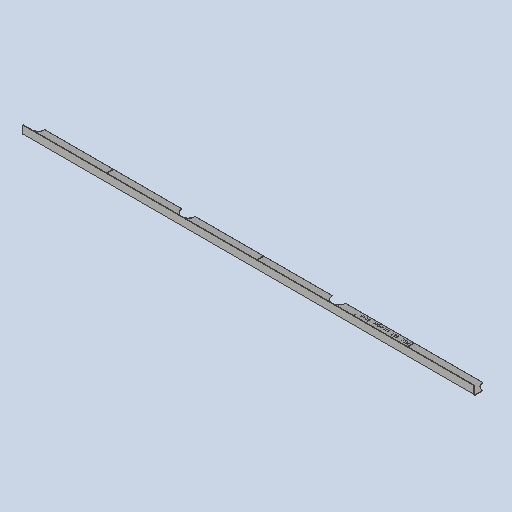
# Autodesk Inventor part: MSC 061 stringer back ^
Saved by Autodesk Inventor 2024.2 (Build 282272000, 272)
## iProperties
Created: 2024-04-28
Part Number: MSC 061 stringer back ^
Material: Stainless Steel
Document SubType Name: Sheet Metal
Designer: pokla
Density: 8 g/cm^3
Sheet Metal Rule: AISI304 2mm Die16
Appearance: Default
Flat Pattern Width: 150 cm
Flat Pattern Length: 7.7967 cm
Flat Pattern Area: 1169.51 cm^2
Sheet Metal Width: 1500,000 mm
Sheet Metal Length: 77,967 mm
Sheet Metal Area: 116950,534 mm^2
Stock Number: МОО 061 стрингер спина ^
Author: admin
Autodesk Inventor part; units mm, degrees
ref_plane "YZ Plane" through (0, 0, 0) normal (1, 0, 0) x (0, 1, 0)
ref_plane "XZ Plane" through (0, 0, 0) normal (0, 1, 0) x (-1, 0, 0)
ref_plane "XY Plane" through (0, 0, 0) normal (0, 0, 1) x (1, 0, 0)
sketch "Sketch1" plane through (0, 0, 0) normal (0, 0, 1) x (1, 0, 0)
  line L0 (-750, 51.765) -> (750, 51.765)
  line L1 (750, 51.765) -> (750, 0)
  line L2 (750, 0) -> (-750, 0)
  line L3 (-750, 0) -> (-750, 51.765)
  point P0 (0, 0)
  point P1 (0, 0)
  dimension "d0" = 1500
  dimension "d1" = 51.765
  measures "d0" distance of L1.end L2.end
  measures "d1" distance of L0.end L1.end
extrude "Plate1" add sketch "Sketch1" along normal blind 2
sketch "Sketch2" plane through (750, 2, 0) normal (0, -1, 0) x (1, 0, 0)
  line L0 (-1500, 0) -> (0, 0)
  line L1 (0, 0) -> (0, 30)
  line L2 (0, 30) -> (-1500, 30)
  line L3 (-1500, 30) -> (-1500, 0)
  constraints: 6 end point, 1 horizontal, 1 perpendicular, 1 vertical
edge flange "Flange1" height 30 angle 90 thickness 2 bend radius 2.75 thickness toward (0, -1, 0) relief round relief width 2 relief depth 1 edges at (0, 0, 2) wall of the first edge with corners at (-750, 2, 0) (750, 2, 0) (750, 2, 30) (-750, 2, 30)
bend "Bend1"
corner "Corner1"
sketch "Sketch5" plane through (0, 0, 0) normal (0, 0, -1) x (-1, 0, 0)
  line L0 (750, 51.765) -> (-750, 51.765) projected
  line L1 (-1, 30) -> (-1, 51.765)
  line L2 (750, 0) -> (-750, 0) projected
  line L3 (-1, 30) -> (1, 30)
  line L4 (1, 30) -> (1, 51.765)
  point P0 (0, 0)
  point P1 (0, 30)
  point P2 (0, 0)
  dimension "d27" = 2
  dimension "d29" = 30
  constraints: 6 end point, 2 midpoint, 2 point on line, 1 horizontal, 1 parallel, 1 perpendicular, 1 vertical alignment
  measures "d27" distance of L1.start L3.end
  measures "d29" distance from line of L2 L3.end
extrude "Extrusion1" cut sketch "Sketch5" against normal through all
pattern_linear "Rectangular Pattern1" count 3 spacing 500 along (1, 0, 0) of "Extrusion1" first direction both ways yes
sketch "Sketch6" plane through (0, 0, 0) normal (0, 0, -1) x (-1, 0, 0)
  line L0 (-750, 51.765) -> (-750, 4.75) projected
  circle A0 centre (-750, 51.765) radius 22.5
  line L1 (-750, 51.765) -> (750, 51.765) projected
  line L2 (-499, 30) -> (-501, 30) construction
  line L3 (-499, 30) -> (-1, 30) construction
  line L4 (-1, 30) -> (-1, 51.765) construction
  line L5 (-1, 51.765) -> (-499, 51.765) projected
  circle A1 centre (-250, 51.765) radius 22.5
  point P0 (0, 0)
  point P1 (-727.5, 51.765)
  point P2 (-750, 29.265)
  point P3 (-250, 30)
  point P4 (-227.5, 51.765)
  point P5 (-272.5, 51.765)
  dimension "d24" = 45
  constraints: 2 centre point, 2 end point, 2 midpoint, 1 equal radius, 1 parallel, 1 vertical alignment
  measures "d24" diameter of A0
extrude "Extrusion2" cut sketch "Sketch6" against normal through all contours L1 A0 L0 | L1 A1 picked at (-748.3311, 36.953) picked at (-248.2369, 40.8343)
mirror "Mirror1" about plane through (0, 0, 0) normal (1, 0, 0) of "Extrusion2"
sketch "Sketch7" plane through (0, 0, 2) normal (0, 0, 1) x (1, 0, 0)
  arc A0 (-750, 29.265) -> (-727.5, 51.765) centre (-750, 51.765) ccw projected
  line L0 (-750, 4.75) -> (-750, 29.265) projected
  line L1 (-750, 4.75) -> (750, 4.75) projected
  line L2 (750, 29.265) -> (750, 4.75) projected
  arc A1 (727.5, 51.765) -> (750, 29.265) centre (750, 51.765) ccw projected
  line L3 (501, 51.765) -> (727.5, 51.765) projected
  line L4 (501, 51.765) -> (501, 30) projected
  line L5 (501, 30) -> (499, 30) projected
  line L6 (499, 30) -> (499, 51.765) projected
  line L7 (1, 51.765) -> (227.5, 51.765) projected
  line L8 (1, 51.765) -> (1, 30) projected
  line L9 (1, 30) -> (-1, 30) projected
  line L10 (-1, 30) -> (-1, 51.765) projected
  line L11 (-499, 51.765) -> (-272.5, 51.765) projected
  line L12 (-499, 51.765) -> (-499, 30) projected
  line L13 (-499, 30) -> (-501, 30) projected
  line L14 (-501, 30) -> (-501, 51.765) projected
  line L15 (-727.5, 51.765) -> (-501, 51.765) projected
  line L16 (649, 50.765) -> (651, 50.765)
  line L17 (651, 50.765) -> (651, 51.765)
  line L18 (651, 51.765) -> (649, 51.765)
  line L19 (649, 51.765) -> (649, 50.765)
  line L20 (650, 4.75) -> (650, 51.765) construction
  line L21 (272.5, 51.765) -> (499, 51.765) projected
  arc A2 (227.5, 51.765) -> (272.5, 51.765) centre (250, 51.765) ccw projected
  line L22 (-227.5, 51.765) -> (-1, 51.765) projected
  arc A3 (-272.5, 51.765) -> (-227.5, 51.765) centre (-250, 51.765) ccw projected
  point P0 (0, 0)
  point P1 (650, 50.765)
  point P2 (649, 51.265)
  point P3 (650, 28.2575)
  dimension "d30" = 2
  dimension "d31" = 1
  dimension "d33" = 100
  constraints: 10 end point, 4 midpoint, 2 parallel, 2 perpendicular, 2 point on line, 1 horizontal, 1 vertical alignment
  measures "d30" distance of L18.end L17.end
  measures "d31" distance of L16.end L17.end
  measures "d33" distance between parallel lines of L20 L2
extrude "Extrusion3" [suppressed]
mirror "Mirror2" [suppressed]
sketch "Sketch9" plane through (0, 0, 2) normal (0, 0, 1) x (1, 0, 0)
  line L0 (494, 46.765) -> (494, 34.765) construction
  line L1 (494, 34.765) -> (294, 34.765) construction
  line L2 (294, 34.765) -> (294, 46.765) construction
  line L3 (294, 46.765) -> (494, 46.765) construction
  line L4 (499, 30) -> (499, 51.765) projected
  line L5 (1, 51.765) -> (499, 51.765) projected
  point P0 (0, 0)
  dimension "d38" = 200
  dimension "d39" = 12
  dimension "d42" = 5
  dimension "d43" = 5
  constraints: 2 other
  measures "d38" distance of L0.end L1.end
  measures "d39" distance of L1.end L2.end
  measures "d42" distance between parallel lines of L4 L0
  measures "d43" distance between parallel lines of L5 L3
mark "Mark3"
equation "\"d1\" = Стрингер_1"
equation "\"d27\" = d18"
equation "\"d29\" = Стрингер_глубина_паза"
equation "\"d43\" = d42"
equation "\"d2\" = Thickness"
equation "\"d3\" = BendReliefWidth"
equation "\"d4\" = BendReliefDepth"
equation "\"d5\" = MinimumRemnant"
equation "\"d6\" = TransitionRadius"
equation "\"d9\" = BendRadius"
equation "\"d10\" = CornerReliefSize"
equation "\"d11\" = GapSize"
equation "\"d12\" = JacobiRadiusSize"
equation "\"BendReliefWidth\" = Thickness"
equation "\"BendReliefDepth\" = 0.5 * Thickness"
equation "\"CornerReliefSize\" = 4 * Thickness"
equation "\"MinimumRemnant\" = 2 * Thickness"
equation "\"TransitionRadius\" = BendRadius"
equation "\"JacobiRadiusSize\" = BendRadius"
equation "\"GapSize\" = Thickness"
equation "\"d18\" = Thickness"
equation "\"qqqqqq\" = 67.35706"
equation "\"Стрингер_1\" = 51.765032"
equation "\"Стрингер_глубина_паза\" = 30"
equation "\"Thickness\" = 2"
equation "\"BendRadius\" = 2.75"
body "Solid1"
